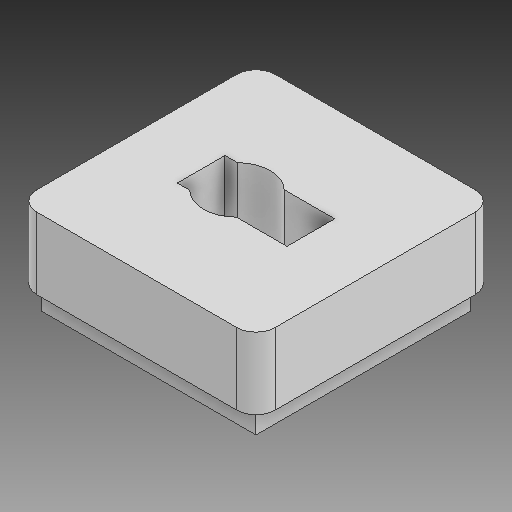
# Autodesk Inventor part: platform
Saved by Autodesk Inventor 2026 (Build 300175000, 175)
## iProperties
Created: 2025-10-18
Part Number: platform
Material: Типовые
Document SubType Name: Modeling
Designer: Admin
Density: 1 g/cm^3
Appearance: По умолчанию
Author: Admin
Autodesk Inventor part; units mm, degrees
ref_plane "YZ Plane" through (0, 0, 0) normal (1, 0, 0) x (0, 1, 0)
ref_plane "XZ Plane" through (0, 0, 0) normal (0, 1, 0) x (-1, 0, 0)
ref_plane "XY Plane" through (0, 0, 0) normal (0, 0, 1) x (1, 0, 0)
sketch "Эскиз1" plane through (0, 0, 0) normal (0, 1, 0) x (-1, 0, 0)
  line L0 (-21, 25) -> (21, 25)
  line L1 (25, 21) -> (25, -21)
  line L2 (21, -25) -> (-21, -25)
  line L3 (-25, -21) -> (-25, 21)
  line L4 (-25, 25) -> (25, -25) construction
  line L5 (25, 25) -> (-25, -25) construction
  line L6 (-11.5, -5) -> (11.5, -5)
  line L7 (11.5, -5) -> (11.5, 5)
  line L8 (11.5, 5) -> (-11.5, 5)
  line L9 (-11.5, 5) -> (-11.5, -5)
  line L10 (-11.5, -5) -> (11.5, 5) construction
  line L11 (11.5, -5) -> (-11.5, 5) construction
  line L12 (-3.5, 5) -> (-3.5, -5)
  line L13 (4, 5) -> (4, -5) construction
  circle A0 centre (4, 0) radius 7.25
  arc A1 (21, -25) -> (25, -21) centre (21, -21) ccw
  arc A2 (25, 21) -> (21, 25) centre (21, 21) ccw
  arc A3 (-21, 25) -> (-25, 21) centre (-21, 21) ccw
  arc A4 (-25, -21) -> (-21, -25) centre (-21, -21) ccw
  point P0 (0, 0)
  point P1 (-1.25, -5)
  point P2 (-1.25, 5)
  dimension "d0" = 50
  dimension "d1" = 50
  dimension "d2" = 23
  dimension "d3" = 10
  dimension "d4" = 8
  dimension "d29" = 7.5
  dimension "d30" = 14.5
  dimension "d52" = 4
  constraints: 28 end point, 12 point on line, 8 point on circle, 8 tangent, 5 centre point, 5 midpoint, 4 parallel, 3 equal radius, 3 perpendicular, 2 horizontal, 1 vertical
  measures "d0" distance of L4.end L5.end
  measures "d1" distance of L5.start L4.end
  measures "d2" distance of L8.end L7.end
  measures "d3" distance of L7.end L6.end
  measures "d4" distance between parallel lines of L9 L12
  measures "d29" distance between parallel lines of L12 L13
  measures "d30" diameter of A0
  measures "d52" radius of A1
extrude "Выдавливание13" add sketch "Эскиз1" along normal blind 15 contours L0 A2 L1 A1 L2 A4 L3 A3 | L6 A0 | A0 L8
sketch "Эскиз6" plane through (0, 0, 0) normal (0, -1, 0) x (1, 0, 0)
  line L0 (22.5, 22.5) -> (-22.5, 22.5)
  line L1 (-22.5, 22.5) -> (-22.5, -22.5)
  line L2 (-22.5, -22.5) -> (22.5, -22.5)
  line L3 (22.5, -22.5) -> (22.5, 22.5)
  line L4 (22.5, 22.5) -> (-22.5, -22.5) construction
  line L5 (-22.5, 22.5) -> (22.5, -22.5) construction
  point P0 (0, 0)
  dimension "d41" = 45
  dimension "d42" = 45
  constraints: 12 end point, 2 midpoint, 2 parallel, 1 horizontal, 1 perpendicular
  measures "d41" distance of L2.end L1.end
  measures "d42" distance of L1.end L0.end
extrude "Выдавливание14" add sketch "Эскиз6" along normal blind 5
extrude "Выдавливание15" cut sketch "Эскиз1" against normal through all contours L12 L8 A0 L6 | A0 L8 L6 | A0 L8 L7 L6
sketch "Эскиз7" plane through (0, 15, 0) normal (0, 1, 0) x (1, 0, 0)
  circle A0 centre (-4.0005, 0) radius 7
  line L0 (21, 25) -> (-21, 25) projected
  line L1 (-25, 21) -> (-25, -21) projected
  point P0 (0, 0)
  point P1 (25, 25)
  point P2 (-25, 25)
  point P3 (-25, -25)
  dimension "d47" = 14
  dimension "d48" = 25
  dimension "d49" = 20.9995
  constraints: 1 centre point
  measures "d47" diameter of A0
  measures "d48" distance from line of L0 A0.centre
  measures "d49" distance from line of L1 A0.centre
extrude "Выдавливание16" cut sketch "Эскиз7" against normal blind 15
sketch "Эскиз8" plane through (0, -5, 0) normal (0, -1, 0) x (1, 0, 0)
  point P0 (0, 0)
sketch "Эскиз9" plane through (0, -5, 0) normal (0, -1, 0) x (1, 0, 0)
  point P0 (0, 0)
sketch "Эскиз10" plane through (0, -5, 0) normal (0, -1, 0) x (1, 0, 0)
  line L0 (-11.5, -7.3) -> (11, -7.3)
  line L1 (11, -7.3) -> (11, 7.3)
  line L2 (11, 7.3) -> (-11.5, 7.3)
  line L3 (-11.5, 7.3) -> (-11.5, -7.3)
  point P0 (0, 0)
  dimension "d53" = 11.5
  dimension "d54" = 14.6
  dimension "d55" = 7.3
  dimension "d56" = 22.5
  constraints: 8 end point, 2 parallel, 1 horizontal, 1 perpendicular
  measures "d53" distance from line of point (0, 0) L3
  measures "d54" distance of L2.end L0.start
  measures "d55" distance from line of point (0, 0) L0
  measures "d56" distance between parallel lines of L3 L1
extrude "Выдавливание17" cut sketch "Эскиз10" against normal blind 1
